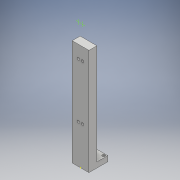
# Autodesk Inventor part: L bracket
Saved by Autodesk Inventor 2017.3 (Build 213256000, 256)
## iProperties
Created: 2017-12-04
Part Number: L bracket
Material: Generic
Document SubType Name: Modeling
Designer: Mac
Density: 1 g/cm^3
Appearance: Default
Author: Mac
Autodesk Inventor part; units mm, degrees
ref_plane "YZ Plane" through (0, 0, 0) normal (1, 0, 0) x (0, 1, 0)
ref_plane "XZ Plane" through (0, 0, 0) normal (0, 1, 0) x (-1, 0, 0)
ref_plane "XY Plane" through (0, 0, 0) normal (0, 0, 1) x (1, 0, 0)
sketch "Sketch1" plane through (0, 0, 0) normal (0, 0, 1) x (1, 0, 0)
  line L0 (-10, -7.525) -> (10, -7.525)
  line L1 (10, -7.525) -> (10, 15)
  line L2 (10, 15) -> (-10, 15)
  line L3 (-10, 15) -> (-10, -7.525)
  point P0 (0, 0)
  dimension "d0" = 20
  dimension "d1" = 22.525
  constraints: 8 end point, 2 parallel, 1 horizontal, 1 perpendicular
  measures "d0" distance of L2.end L1.end
  measures "d1" distance of L1.end L0.end
extrude "Extrusion1" add sketch "Sketch1" along normal blind 6.35
sketch "Sketch2" plane through (0, 0, 6.35) normal (0, 0, 1) x (1, 0, 0)
  line L0 (-10, -7.525) -> (10, -7.525) projected
  line L1 (10, -7.525) -> (10, 15) projected
  line L2 (-10, -7.525) -> (10, -7.525)
  line L3 (10, -7.525) -> (10, -1.175)
  line L4 (10, -1.175) -> (-10, -1.175)
  line L5 (-10, -1.175) -> (-10, -7.525)
  point P0 (0, 0)
  constraints: 8 end point, 2 parallel, 1 horizontal, 1 perpendicular, 1 point on line
extrude "Extrusion2" add sketch "Sketch2" along normal blind 120
sketch "Sketch4" plane through (0, 0, 6.35) normal (0, 0, 1) x (1, 0, 0)
  point P0 (0, 0)
  point P1 (-7.5, 12.5)
  point P2 (7.5, 12.5)
hole "Hole2" at (-7.5, 12.5, 6.35) at (7.5, 12.5, 6.35) direction (0, 0, -1) diameter 3.175 depth 12 tip angle 118
sketch "Sketch5" plane through (-10, -1.175, 6.35) normal (0, 1, 0) x (1, 0, 0)
  line L0 (20, 6.35) -> (20, -120) projected
  line L1 (0, 26.05) -> (20, 26.05)
  line L2 (20, 26.05) -> (20, -120)
  line L3 (20, -120) -> (0, -120)
  line L4 (0, -120) -> (0, 26.05)
  point P0 (10, 6.35)
  constraints: 8 end point, 2 parallel, 1 horizontal, 1 perpendicular
extrude "Extrusion3" add sketch "Sketch5" along normal blind 3.175
sketch "Sketch6" plane through (-10, -7.525, 0) normal (0, -1, 0) x (1, 0, 0)
  point P0 (10, 0)
  point P1 (12.5, 149.5)
  point P2 (7.5, 149.5)
sketch "Sketch7" plane through (-10, 2, 6.35) normal (0, 1, 0) x (1, 0, 0)
  point P0 (10, 6.35)
  point P1 (7.5, -105)
  point P2 (12.5, -105)
hole "Hole5" at (-2.5, 2, 111.35) at (2.5, 2, 111.35) direction (0, -1, 0) diameter 3.175 depth 16.265 tip angle 118
pattern_linear "Rectangular Pattern4" count 2 spacing 65 along (0, 0, -1) of "Hole5"
sketch "Sketch8" plane through (10, -1.175, -19.7) normal (0, 0, -1) x (-1, 0, 0)
  line L0 (-3.9221, 5.4444) -> (30.2334, 5.4444)
  line L1 (30.2334, 5.4444) -> (30.2334, -5.6932)
  line L2 (30.2334, -5.6932) -> (-3.9221, -5.6932)
  line L3 (-3.9221, -5.6932) -> (-3.9221, 5.4444)
  point P0 (10, 1.175)
  constraints: 8 end point, 2 parallel, 1 horizontal, 1 perpendicular
extrude "Extrusion4" cut sketch "Sketch8" against normal blind 19.7
body "Solid1"
